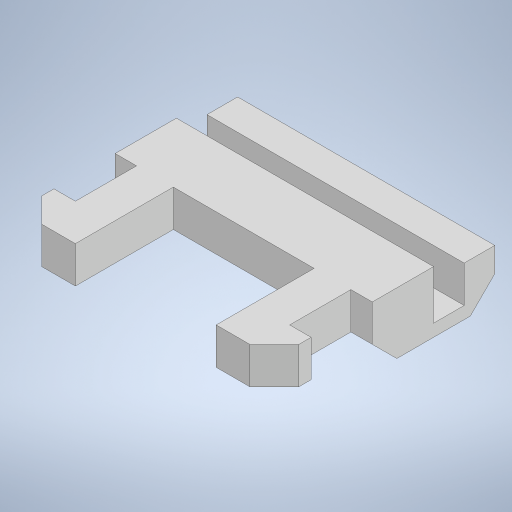
# Autodesk Inventor part: Breakout Clip
Saved by Autodesk Inventor 2024.1 (Build 281209000, 209)
## iProperties
Created: 2024-02-02
Part Number: Breakout Clip
Material: Generic
Document SubType Name: Modeling
Designer: ryanm
Density: 1 g/cm^3
Appearance: Default
Author: ryanm
Autodesk Inventor part; units mm, degrees
ref_plane "YZ Plane" through (0, 0, 0) normal (1, 0, 0) x (0, 1, 0)
ref_plane "XZ Plane" through (0, 0, 0) normal (0, 1, 0) x (-1, 0, 0)
ref_plane "XY Plane" through (0, 0, 0) normal (0, 0, 1) x (1, 0, 0)
sketch "Sketch1" plane through (0, 0, 0) normal (0, 1, 0) x (-1, 0, 0)
  line L0 (10.5, -9) -> (-10.5, -9)
  line L1 (-10.5, -9) -> (-10.5, 9)
  line L2 (-10.5, 9) -> (10.5, 9)
  line L3 (10.5, 9) -> (10.5, -9)
  point P0 (0, 0)
  point P1 (0, -9)
  point P2 (10.5, 0)
  dimension "d0" = 21
  dimension "d1" = 18
  constraints: 8 end point, 2 midpoint, 2 parallel, 1 horizontal, 1 horizontal alignment, 1 perpendicular, 1 vertical alignment
  measures "d0" distance of L0.start L0.end
  measures "d1" distance of L2.end L0.start
extrude "Extrusion1" add sketch "Sketch1" along normal blind 5
sketch "Sketch2" plane through (-10.5, 0, -9) normal (-1, 0, 0) x (0, 0, 1)
  line L0 (18, 0) -> (10, 0)
  line L1 (10, 0) -> (10, 2)
  line L2 (10, 2) -> (18, 2)
  line L3 (18, 2) -> (18, 0)
  point P0 (9, 0)
  dimension "d4" = 2
  dimension "d5" = 8
  constraints: 8 end point, 2 parallel, 1 horizontal, 1 perpendicular
  measures "d4" distance of L0.end L1.end
  measures "d5" distance of L1.end L2.end
extrude "Extrusion2" cut sketch "Sketch2" against normal through all
sketch "Sketch3" plane through (-10.5, 2, 1) normal (0, -1, 0) x (1, 0, 0)
  line L0 (21, 8) -> (21, -10) projected
  line L1 (21, 0) -> (19.25, 0)
  line L2 (19.25, 0) -> (19.25, 5)
  line L3 (19.25, 5) -> (21, 5)
  line L4 (21, 5) -> (21, 0)
  line L5 (0, -10) -> (0, 8) projected
  line L6 (0, 0) -> (1.75, 0)
  line L7 (1.75, 0) -> (1.75, 5)
  line L8 (1.75, 5) -> (0, 5)
  line L9 (0, 5) -> (0, 0)
  line L10 (0, 8) -> (21, 8) projected
  point P0 (10.5, -1)
  point P1 (0, 5)
  dimension "d8" = 5
  dimension "d9" = 3
  dimension "d10" = 17.5
  constraints: 16 end point, 4 parallel, 2 equal length, 2 horizontal, 2 perpendicular, 2 point on line, 1 horizontal alignment
  measures "d8" distance of L1.end L2.end
  measures "d9" distance between parallel lines of L10 L3
  measures "d10" distance between parallel lines of L7 L2
extrude "Extrusion3" cut sketch "Sketch3" against normal through all
sketch "Sketch4" plane through (-10.5, 2, 9) normal (0, -1, 0) x (1, 0, 0)
  line L0 (16.25, -8) -> (4.75, -8)
  line L1 (4.75, -8) -> (4.75, 0)
  line L2 (4.75, 0) -> (16.25, 0)
  line L3 (16.25, 0) -> (16.25, -8)
  line L4 (19.25, -8) -> (19.25, -3) projected
  line L5 (1.75, -3) -> (1.75, -8) projected
  point P0 (10.5, -9)
  point P1 (21, 0)
  point P2 (0, -8)
  dimension "d13" = 3
  dimension "d14" = 3
  constraints: 8 end point, 2 horizontal alignment, 2 parallel, 1 horizontal, 1 perpendicular
  measures "d13" distance between parallel lines of L3 L4
  measures "d14" distance between parallel lines of L5 L1
extrude "Extrusion4" cut sketch "Sketch4" against normal through all
chamfer "Chamfer1" distance 2 angle 45 2 edges at (10.5, 3.5, 9) (-10.5, 3.5, 9)
sketch "Sketch6" plane through (-10.5, 0, -9) normal (-1, 0, 0) x (0, 0, 1)
  line L0 (10, 5) -> (0, 5) projected
  line L1 (2.5, 5) -> (5, 5)
  line L2 (5, 5) -> (5, 1)
  line L3 (5, 1) -> (2.5, 1)
  line L4 (2.5, 1) -> (2.5, 5)
  line L5 (0, 0) -> (10, 0) projected
  line L6 (10, 0) -> (10, 5) projected
  point P0 (9, 0)
  dimension "d20" = 2.5
  dimension "d22" = 1
  dimension "d23" = 5
  constraints: 8 end point, 2 parallel, 1 horizontal, 1 perpendicular, 1 point on line
  measures "d20" distance of L2.end L3.end
  measures "d22" distance between parallel lines of L5 L3
  measures "d23" distance between parallel lines of L6 L2
extrude "Extrusion5" cut sketch "Sketch6" against normal through all
chamfer "Chamfer2" distance 2 angle 45 2 edges at (0, 0, 1) (0, 0, -9)
sketch "Sketch7" plane through (10.5, 1, -6.5) normal (1, 0, 0) x (0, 0, -1)
  line L0 (0, 4) -> (0, 0) projected
  line L1 (0, 4) -> (2.5, 4) projected
  line L2 (2.5, 1) -> (2.5, 4) projected
  line L3 (2.5, 3) -> (0, 3)
  point P0 (-6.5, -1)
  dimension "d30" = 1
  constraints: 2 end point, 2 point on line, 1 perpendicular
  measures "d30" distance between parallel lines of L1 L3
extrude "Extrusion6" cut sketch "Sketch7" against normal through all
equation "\"d14\" = d13"
body "Solid1"
